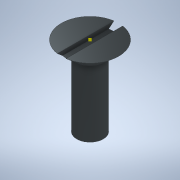
# Autodesk Inventor part: tornillo corto f
Saved by Autodesk Inventor 2020.3 (Build 243373000, 373)
## iProperties
Created: 2020-10-13
Part Number: tornillo corto f
Material: Hierro, fundido
Document SubType Name: Modeling
Designer: HUAWEI
Density: 7.15 g/cm^3
Appearance: Gris hierro
Author: HUAWEI
Autodesk Inventor part; units mm, degrees
ref_plane "YZ Plane" through (0, 0, 0) normal (1, 0, 0) x (0, 1, 0)
ref_plane "XZ Plane" through (0, 0, 0) normal (0, 1, 0) x (-1, 0, 0)
ref_plane "XY Plane" through (0, 0, 0) normal (0, 0, 1) x (1, 0, 0)
sketch "Boceto1" plane through (0, 0, 0) normal (0, 0, 1) x (1, 0, 0)
  line L0 (0, -18) -> (3, -18)
  line L1 (3, -18) -> (3, -3)
  line L2 (0, 0) -> (6.5, 0)
  line L3 (3, -3) -> (6.5, 0)
  line L4 (0, 2.8182) -> (0, -20.4465)
  line L5 (0, 0) -> (0, -1)
  dimension "d0" = 3
  dimension "d1" = 15
  dimension "d2" = 6.5
  dimension "d3" = 3
  dimension "d4" = 0
  dimension "d5" = 1
  constraints: 12 end point, 2 horizontal, 1 perpendicular, 1 point on line, 1 vertical
  measures "d0" distance of L0.start L0.end
  measures "d1" distance of L0.end L1.end
  measures "d2" distance of L2.start L2.end
  measures "d3" distance from line of L2 L1.end
  measures "d4" distance from line of point (0, 0) L2
  measures "d5" distance of L2.start L5.end
revolve "Revolución1" add sketch "Boceto1" angle 360 about axis through (0, 2.8182, 0) along (0, -1, 0)
sketch "Boceto2" plane through (0, 0, 0) normal (0, 0, 1) x (1, 0, 0)
  line L0 (0, 0) -> (1, 0)
  line L1 (-6.5, 0) -> (6.5, 0) projected
  line L2 (1, 0) -> (1, -1)
  line L3 (1, -1) -> (0, -1)
  line L4 (1, -1) -> (-1, -1)
  line L5 (-1, -1) -> (-1, 0)
  dimension "d7" = 1
  dimension "d8" = 1
  dimension "d10" = 2
  constraints: 10 end point, 3 perpendicular, 2 point on line, 1 horizontal
  measures "d7" distance of L0.start L0.end
  measures "d8" distance of L0.end L2.end
  measures "d10" distance of L2.end L4.end
extrude "Extrusión1" cut sketch "Boceto2" along normal mid plane 15
sketch "Boceto3" plane through (0, 0, 0) normal (0, 0, 1) x (1, 0, 0)
  point P0 (0, 0)
sketch "Boceto4" plane through (0, 0, 0) normal (0, 0, 1) x (1, 0, 0)
  line L0 (-3, -18) -> (3, -18) projected
  line L1 (3, -18) -> (0, -19.7321)
  line L2 (0, -19.7321) -> (0, -18)
  point P0 (0, 0)
  constraints: 4 end point, 1 midpoint
revolve "Revolución2" add sketch "Boceto4" angle 360 about axis through (0, -19.7321, 0) along (0, 1, 0)
